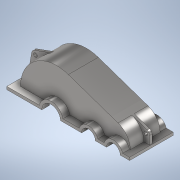
# Autodesk Inventor part: МПСТ Крышка корпуса
Saved by Autodesk Inventor 2022.1 (Build 261234020, 234B)
## iProperties
Created: 2021-12-09
Part Number: МПСТ Крышка корпуса
Material: Сталь, углеродистая
Document SubType Name: Modeling
Designer: Алексанян Г.
Density: 7.85 g/cm^3
Appearance: С умеренной полировкой
Author: Алексанян Г.
Autodesk Inventor part; units mm, degrees
ref_plane "XZ Plane" through (0, 0, 0) normal (0, 1, 0) x (-1, 0, 0)
ref_plane "XY Plane" through (0, 0, 0) normal (0, 0, 1) x (1, 0, 0)
sketch "Эскиз1" plane through (0, 0, 0) normal (0, 1, 0) x (-1, 0, 0)
  line L0 (493, -175) -> (-493, -175)
  line L1 (-493, -175) -> (-493, 175)
  line L2 (-493, 175) -> (493, 175)
  line L3 (493, 175) -> (493, -175)
  line L4 (493, -175) -> (-493, 175) construction
  line L5 (-493, -175) -> (493, 175) construction
  point P0 (0, 0)
  dimension "d0" = 350
  dimension "d1" = 986
  constraints: 12 end point, 2 midpoint, 2 parallel, 1 horizontal, 1 perpendicular
  measures "d0" distance of L0.end L1.end
  measures "d1" distance of L0.start L0.end
extrude "Выдавливание1" add sketch "Эскиз1" along normal blind 22.5
sketch "Эскиз2" plane through (0, 0, 0) normal (0, 0, 1) x (1, 0, 0)
  line L0 (493, 22.5) -> (-493, 22.5) projected
  arc A0 (-53.7175, 296.7459) -> (-438, 22.5) centre (-148, 22.5) ccw
  line L1 (-53.7175, 296.7459) -> (345.1413, 159.6229)
  arc A1 (443, 22.5) -> (345.1413, 159.6229) centre (298, 22.5) ccw
  point P0 (0, 0)
  dimension "d4" = 290
  dimension "d5" = 145
  dimension "d6" = 50
  dimension "d7" = 55
  constraints: 4 point on circle, 4 point on line, 2 centre point, 2 end point, 2 tangent
  measures "d4" radius of A0
  measures "d5" radius of A1
  measures "d6" distance of L0.start A1.start
  measures "d7" distance of L0.end A0.end
extrude "Выдавливание2" add sketch "Эскиз2" along normal mid plane 240
shell "Оболочка1" thickness 6 removed faces 1 at (-164.3333, 0, 58.3333)
sketch "Эскиз3" plane through (-487, 16.5, 169) normal (0, -1, 0) x (1, 0, 0)
  line L0 (55.0634, -283) -> (923.8704, -283) projected
  line L1 (55.0634, -55) -> (55.0634, -283) projected
  line L2 (923.8704, -55) -> (55.0634, -55) projected
  line L3 (923.8704, -283) -> (923.8704, -55) projected
  line L4 (0, 0) -> (974, 0) projected
  line L5 (0, -338) -> (0, 0) projected
  line L6 (974, -338) -> (0, -338) projected
  line L7 (974, 0) -> (974, -338) projected
  point P0 (487, -169)
extrude "Выдавливание3" add sketch "Эскиз3" along normal up to surface (16.5 mm away)
sketch "Эскиз4" plane through (-493, 0, 175) normal (0, 0, 1) x (1, 0, 0)
  line L0 (0, 0) -> (986, 0) projected
  circle A0 centre (856, 0) radius 55
  circle A1 centre (656, 0) radius 55
  circle A2 centre (356, 0) radius 75
  circle A3 centre (356, 0) radius 97.5
  circle A4 centre (656, 0) radius 77.5
  circle A5 centre (856, 0) radius 77.5
  point P0 (493, 0)
  point P1 (493, 0)
  point P2 (933.5, 0)
  point P3 (778.5, 0)
  point P4 (801, 0)
  point P5 (911, 0)
  point P6 (733.5, 0)
  point P7 (578.5, 0)
  point P8 (601, 0)
  point P9 (711, 0)
  point P10 (453.5, 0)
  point P11 (258.5, 0)
  point P12 (281, 0)
  point P13 (431, 0)
  dimension "d13" = 130
  dimension "d14" = 200
  dimension "d15" = 300
  dimension "d16" = 110
  dimension "d17" = 110
  dimension "d18" = 150
  dimension "d19" = 22.5
  dimension "d20" = 22.5
  dimension "d21" = 22.5
  constraints: 6 centre point, 3 coincident, 3 horizontal alignment, 1 midpoint
  measures "d13" distance of L0.end point (856, 0)
  measures "d14" distance of point (656, 0) point (856, 0)
  measures "d15" distance of point (356, 0) point (656, 0)
  measures "d16" diameter of A0
  measures "d17" diameter of A1
  measures "d18" diameter of A2
  measures "d19" radial gap between concentric circles of A2 A3
  measures "d20" radial gap between concentric circles of A1 A4
  measures "d21" radial gap between concentric circles of A0 A5
extrude "Выдавливание4" add sketch "Эскиз4" against normal up to surface (55 mm away) contours A2 L0 A3 | A1 L0 A4 | A0 L0 A5 picked at (266.3308, 4.6252) picked at (620.9156, 60.3286) picked at (820.9156, 60.3286)
extrude "Выдавливание5" cut sketch "Эскиз4" against normal up to surface (61 mm away) contours L0 A2 | L0 A1 | L0 A0 picked at (372.7619, 29.314) picked at (671.8995, 13.02) picked at (871.8995, 13.02)
sketch "Эскиз5" plane through (493, 0, -175) normal (0, 0, -1) x (-1, 0, 0)
  line L0 (0, 0) -> (986, 0) projected
  circle A0 centre (130, 0) radius 55
  circle A1 centre (330, 0) radius 75
  circle A2 centre (630, 0) radius 75
  circle A3 centre (130, 0) radius 77.5
  circle A4 centre (330, 0) radius 97.5
  circle A5 centre (630, 0) radius 97.5
  point P0 (493, 0)
  point P1 (493, 0)
  point P2 (727.5, 0)
  point P3 (532.5, 0)
  point P4 (555, 0)
  point P5 (705, 0)
  point P6 (427.5, 0)
  point P7 (232.5, 0)
  point P8 (255, 0)
  point P9 (405, 0)
  point P10 (207.5, 0)
  point P11 (52.5, 0)
  point P12 (75, 0)
  point P13 (185, 0)
  dimension "d26" = 130
  dimension "d27" = 200
  dimension "d28" = 300
  dimension "d29" = 110
  dimension "d30" = 150
  dimension "d31" = 150
  dimension "d32" = 22.5
  dimension "d33" = 22.5
  dimension "d34" = 22.5
  constraints: 6 centre point, 3 coincident, 3 horizontal alignment, 1 midpoint
  measures "d26" distance of L0.start point (130, 0)
  measures "d27" distance of point (130, 0) point (330, 0)
  measures "d28" distance of point (330, 0) point (630, 0)
  measures "d29" diameter of A0
  measures "d30" diameter of A1
  measures "d31" diameter of A2
  measures "d32" radial gap between concentric circles of A0 A3
  measures "d33" radial gap between concentric circles of A1 A4
  measures "d34" radial gap between concentric circles of A2 A5
extrude "Выдавливание6" add sketch "Эскиз5" against normal up to surface (55 mm away) contours A0 L0 A3 | A1 L0 A4 | A2 L0 A5 picked at (94.9156, 60.3286) picked at (240.3308, 4.6252) picked at (540.3308, 4.6252)
extrude "Выдавливание7" cut sketch "Эскиз5" against normal up to surface (61 mm away) contours L0 A0 | L0 A1 | L0 A2 picked at (143.5485, 12.3511) picked at (346.7619, 29.314) picked at (650.2254, 14.6946)
sketch "Эскиз6" plane through (0, 0, 0) normal (0, 0, 1) x (1, 0, 0)
  line L0 (493, 22.5) -> (437.162, 22.5) projected
  line L1 (488, 22.5) -> (488, 89.1001)
  line L2 (-53.7175, 296.7459) -> (345.1413, 159.6229) projected
  line L3 (345.1413, 159.6229) -> (467.7534, 117.4703)
  arc A0 (488, 89.1001) -> (467.7534, 117.4703) centre (458, 89.1001) ccw
  arc A1 (443, 22.5) -> (345.1413, 159.6229) centre (298, 22.5) ccw projected
  line L4 (-231.8683, 22.5) -> (-493, 22.5) projected
  line L5 (-488, 22.5) -> (-457.5055, 195.4426)
  arc A2 (-53.7175, 296.7459) -> (-438, 22.5) centre (-148, 22.5) ccw projected
  line L6 (-493, 0) -> (-493, 22.5) projected
  line L7 (-438.2219, 218.424) -> (-302.8556, 267.6933)
  arc A3 (-438.2219, 218.424) -> (-457.5055, 195.4426) centre (-427.9613, 190.2332) ccw
  circle A4 centre (-427.9613, 190.2332) radius 15
  circle A5 centre (458, 89.1001) radius 15
  point P0 (0, 0)
  point P1 (-454.4979, 212.5)
  dimension "d39" = 5
  dimension "d40" = 30
  dimension "d41" = 5
  dimension "d42" = 80
  dimension "d44" = 190
  dimension "d45" = 120
  dimension "d46" = 30
  dimension "d47" = 30
  dimension "d48" = 30
  constraints: 8 end point, 5 point on circle, 4 centre point, 4 point on line, 4 tangent, 2 coincident, 1 collinear, 1 vertical
  measures "d39" distance from line of L0.start L1
  measures "d40" radius of A0
  measures "d41" distance from line of L6 L5.start
  measures "d42" angle of L4 L5
  measures "d44" vertical distance of L5.start point (-454.498, 212.5)
  measures "d45" angle of L5 L7
  measures "d46" radius of A3
  measures "d47" diameter of A4
  measures "d48" diameter of A5
extrude "Выдавливание8" add sketch "Эскиз6" along normal mid plane 20
sketch "Эскиз7" plane through (-493, 0, 175) normal (0, 0, 1) x (1, 0, 0)
  arc A0 (431, 0) -> (281, 0) centre (356, 0) ccw projected
  arc A1 (711, 0) -> (601, 0) centre (656, 0) ccw projected
  point P0 (493, 0)
  constraints: 2 coincident
ref_plane "РабПлоскость2" through (163, 0, 175) normal (1, 0, 0) x (0, 1, 0)
ref_plane "РабПлоскость1" through (-137, 0, 175) normal (1, 0, 0) x (0, 1, 0)
